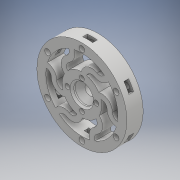
# Autodesk Inventor part: sea_ninjaflex
Saved by Autodesk Inventor 2018 (Build 220112000, 112)
## iProperties
Created: 2019-05-27
Part Number: sea_ninjaflex
Material: Generic
Document SubType Name: Modeling
Designer: Jasper
Mass: 17.2372 g
Surface Area: 57.8706 cm^2
Volume: 17.2372 cm^3
Density: 1 g/cm^3
Appearance: Default
Author: Jasper
Autodesk Inventor part; units mm, degrees
ref_plane "YZ Plane" through (0, 0, 0) normal (1, 0, 0) x (0, 1, 0)
ref_plane "XZ Plane" through (0, 0, 0) normal (0, 1, 0) x (-1, 0, 0)
sketch "Sketch1" plane through (0, 0, 0) normal (0, 1, 0) x (-1, 0, 0)
  circle A0 centre (0, 0) radius 25
  dimension "d0" = 50
  constraints: 1 centre point, 1 coincident
  measures "d0" diameter of A0
extrude "Extrusion1" add sketch "Sketch1" along normal blind 9
sketch "Sketch2" plane through (0, 9, 0) normal (0, 1, 0) x (1, 0, 0)
  line L0 (0, 0) -> (0, -22) construction
  line L1 (0, 0) -> (22, 0) construction
  circle A0 centre (0, -22) radius 1.6
  circle A1 centre (19.0526, -11) radius 1.6
  circle A2 centre (19.0526, 11) radius 1.6
  circle A3 centre (0, 22) radius 1.6
  circle A4 centre (-19.0526, 11) radius 1.6
  circle A5 centre (-19.0526, -11) radius 1.6
  dimension "d3" = 22
  dimension "d4" = 90
  dimension "d5" = 3.2
  dimension "d8" = 360
  constraints: 6 centre point, 4 end point, 1 coincident, 1 horizontal, 1 perpendicular, 1 vertical, 13 other
  measures "d3" distance of L0.start L0.end
  measures "d4" angle of L0 L1
  measures "d5" diameter of A0
extrude "Extrusion2" cut sketch "Sketch2" against normal up to surface (9 mm away)
ref_plane "Work Plane1" through (0, 3.2, 0) normal (0, 1, 0) x (1, 0, 0)
sketch "Sketch3" plane through (0, 3.2, 0) normal (0, 1, 0) x (1, 0, 0)
  circle A0 centre (-19.0526, 11) radius 1.6 construction
  circle A1 centre (-19.0526, -11) radius 1.6 construction
  circle A2 centre (0, 22) radius 1.6 construction
  circle A3 centre (19.0526, -11) radius 1.6 construction
  circle A4 centre (0, -22) radius 1.6 construction
  circle A5 centre (19.0526, 11) radius 1.6 construction
  circle A6 centre (0, 0) radius 25 construction
  line L0 (0, -25.2332) -> (-2.8, -23.6166)
  line L1 (-2.8, -23.6166) -> (-2.8, -20.3834)
  line L2 (-2.8, -20.3834) -> (0, -18.7668)
  line L3 (0, -18.7668) -> (2.8, -20.3834)
  line L4 (2.8, -20.3834) -> (2.8, -23.6166)
  line L5 (2.8, -23.6166) -> (0, -25.2332)
  line L6 (0, 0) -> (0, -18.7668)
  line L7 (0, 0) -> (18.7668, 0) construction
  line L8 (-2.8, -23.6166) -> (2.8, -23.6166)
  line L9 (2.8, -23.6166) -> (2.8, -26)
  line L10 (2.8, -26) -> (-2.8, -26)
  line L11 (-2.8, -26) -> (-2.8, -23.6166)
  line L12 (19.0526, -7.7668) -> (21.8526, -9.3834)
  line L13 (16.2526, -9.3834) -> (19.0526, -7.7668)
  line L14 (21.8526, -9.3834) -> (23.9167, -10.5751)
  line L15 (16.2526, -12.6166) -> (16.2526, -9.3834)
  line L16 (19.0526, -14.2332) -> (21.8526, -9.3834)
  line L17 (21.8526, -12.6166) -> (19.0526, -14.2332)
  line L18 (21.1167, -15.4249) -> (19.0526, -14.2332)
  line L19 (23.9167, -10.5751) -> (21.1167, -15.4249)
  line L20 (21.8526, -9.3834) -> (21.8526, -12.6166)
  line L21 (19.0526, -14.2332) -> (16.2526, -12.6166)
  line L22 (16.2526, 12.6166) -> (19.0526, 14.2332)
  line L23 (16.2526, 9.3834) -> (16.2526, 12.6166)
  line L24 (19.0526, 14.2332) -> (21.1167, 15.4249)
  line L25 (19.0526, 7.7668) -> (16.2526, 9.3834)
  line L26 (21.8526, 9.3834) -> (19.0526, 14.2332)
  line L27 (21.8526, 12.6166) -> (21.8526, 9.3834)
  line L28 (23.9167, 10.5751) -> (21.8526, 9.3834)
  line L29 (21.1167, 15.4249) -> (23.9167, 10.5751)
  line L30 (19.0526, 14.2332) -> (21.8526, 12.6166)
  line L31 (21.8526, 9.3834) -> (19.0526, 7.7668)
  line L32 (-2.8, 20.3834) -> (-2.8, 23.6166)
  line L33 (0, 18.7668) -> (-2.8, 20.3834)
  line L34 (-2.8, 23.6166) -> (-2.8, 26)
  line L35 (2.8, 20.3834) -> (0, 18.7668)
  line L36 (2.8, 23.6166) -> (-2.8, 23.6166)
  line L37 (0, 25.2332) -> (2.8, 23.6166)
  line L38 (2.8, 26) -> (2.8, 23.6166)
  line L39 (-2.8, 26) -> (2.8, 26)
  line L40 (-2.8, 23.6166) -> (0, 25.2332)
  line L41 (2.8, 23.6166) -> (2.8, 20.3834)
  line L42 (-19.0526, 7.7668) -> (-21.8526, 9.3834)
  line L43 (-16.2526, 9.3834) -> (-19.0526, 7.7668)
  line L44 (-21.8526, 9.3834) -> (-23.9167, 10.5751)
  line L45 (-16.2526, 12.6166) -> (-16.2526, 9.3834)
  line L46 (-19.0526, 14.2332) -> (-21.8526, 9.3834)
  line L47 (-21.8526, 12.6166) -> (-19.0526, 14.2332)
  line L48 (-21.1167, 15.4249) -> (-19.0526, 14.2332)
  line L49 (-23.9167, 10.5751) -> (-21.1167, 15.4249)
  line L50 (-21.8526, 9.3834) -> (-21.8526, 12.6166)
  line L51 (-19.0526, 14.2332) -> (-16.2526, 12.6166)
  line L52 (-16.2526, -12.6166) -> (-19.0526, -14.2332)
  line L53 (-16.2526, -9.3834) -> (-16.2526, -12.6166)
  line L54 (-19.0526, -14.2332) -> (-21.1167, -15.4249)
  line L55 (-19.0526, -7.7668) -> (-16.2526, -9.3834)
  line L56 (-21.8526, -9.3834) -> (-19.0526, -14.2332)
  line L57 (-21.8526, -12.6166) -> (-21.8526, -9.3834)
  line L58 (-23.9167, -10.5751) -> (-21.8526, -9.3834)
  line L59 (-21.1167, -15.4249) -> (-23.9167, -10.5751)
  line L60 (-19.0526, -14.2332) -> (-21.8526, -12.6166)
  line L61 (-21.8526, -9.3834) -> (-19.0526, -7.7668)
  point P0 (19.0526, 11)
  point P1 (0, 22)
  point P2 (-19.0526, 11)
  dimension "d13" = 5.6
  dimension "d14" = 90
  dimension "d15" = 5.6
  dimension "d16" = 2.3834
  dimension "d19" = 360
  constraints: 124 end point, 2 horizontal, 2 parallel, 2 perpendicular, 1 coincident, 134 other
  measures "d13" distance between parallel lines of L3 L0
  measures "d14" angle of L6 L7
  measures "d15" distance of L9.end L10.end
  measures "d16" distance between parallel lines of L10 L8
extrude "Extrusion3" cut sketch "Sketch3" along normal blind 2.6
sketch "Sketch4" plane through (0, 9, 0) normal (0, 1, 0) x (1, 0, 0)
  line L0 (0, 0) -> (8, 0) construction
  line L1 (0, 0) -> (8, 0) construction
  circle A0 centre (8, 0) radius 1.35
  circle A1 centre (0, 8) radius 1.35
  circle A2 centre (-8, 0) radius 1.35
  circle A3 centre (0, -8) radius 1.35
  dimension "d23" = 8
  dimension "d24" = 0
  dimension "d25" = 2.7
  dimension "d28" = 360
  constraints: 4 centre point, 4 end point, 2 horizontal, 1 coincident, 1 collinear, 9 other
  measures "d23" distance of L0.start L0.end
  measures "d24" distance between parallel lines of L0 L1
  measures "d25" diameter of A0
extrude "Extrusion4" cut sketch "Sketch4" against normal up to surface (9 mm away)
sketch "Sketch5" plane through (0, 9, 0) normal (0, 1, 0) x (1, 0, 0)
  circle A0 centre (-8, 0) radius 1.35 construction
  circle A1 centre (0, -8) radius 1.35 construction
  circle A2 centre (0, 8) radius 1.35 construction
  circle A3 centre (8, 0) radius 1.35 construction
  circle A4 centre (-19.0526, 11) radius 1.6 construction
  circle A5 centre (-19.0526, -11) radius 1.6 construction
  circle A6 centre (0, 22) radius 1.6 construction
  circle A7 centre (19.0526, -11) radius 1.6 construction
  circle A8 centre (0, -22) radius 1.6 construction
  circle A9 centre (19.0526, 11) radius 1.6 construction
  circle A10 centre (0, 0) radius 25 construction
  circle A11 centre (0, 8) radius 2.25
  circle A12 centre (-8, 0) radius 2.25
  circle A13 centre (0, -8) radius 2.25
  circle A14 centre (8, 0) radius 2.25
  dimension "d32" = 4.5
  dimension "d35" = 360
  constraints: 4 centre point, 1 coincident, 9 other
  measures "d32" diameter of A11
extrude "Extrusion5" cut sketch "Sketch5" against normal blind 5.5
sketch "Sketch6" plane through (0, 9, 0) normal (0, 1, 0) x (1, 0, 0)
  circle A0 centre (0, 0) radius 11
  dimension "d39" = 22
  constraints: 1 centre point, 1 coincident
  measures "d39" diameter of A0
extrude "Extrusion6" [suppressed]
sketch "Sketch7" plane through (0, 9, 0) normal (0, 1, 0) x (1, 0, 0)
  circle A0 centre (0, 0) radius 17.5 construction
  circle A1 centre (0, 0) radius 12.5 construction
  circle A2 centre (0, -8) radius 2.25 construction
  circle A3 centre (0, 8) radius 2.25 construction
  circle A4 centre (-8, 0) radius 2.25 construction
  circle A5 centre (8, 0) radius 2.25 construction
  circle A6 centre (-19.0526, 11) radius 1.6 construction
  circle A7 centre (-19.0526, -11) radius 1.6 construction
  circle A8 centre (0, 22) radius 1.6 construction
  circle A9 centre (19.0526, -11) radius 1.6 construction
  circle A10 centre (0, -22) radius 1.6 construction
  circle A11 centre (19.0526, 11) radius 1.6 construction
  circle A12 centre (0, 0) radius 25 construction
  line L0 (0.0443, -12.4999) -> (-1.2042, -12.4373)
  line L1 (0.0443, -12.4999) -> (1.2943, -12.4999) construction
  line L2 (0.0443, -12.4999) -> (1.2927, -12.4373)
  line L3 (0.0443, -12.4999) -> (1.2943, -12.4999) construction
  line L4 (-1.2042, -12.4373) -> (3.5115, -17.153)
  line L5 (-1.2042, -12.4373) -> (5.4648, -12.4373) construction
  line L6 (1.2796, -12.4428) -> (5.4791, -16.6424)
  line L7 (1.2796, -12.4428) -> (7.2186, -12.4428) construction
  arc A13 (-1.1991, -12.4423) -> (1.2796, -12.4428) centre (0.0427, -0.0042) ccw
  arc A14 (3.5115, -17.153) -> (5.4791, -16.6424) centre (0.1064, 0.0125) ccw
  line L8 (3.6487, -11.9681) -> (9.8101, -14.5202)
  arc A15 (3.6553, -11.9708) -> (5.9455, -11.0227) centre (0.0427, -0.0042) ccw
  line L9 (5.9455, -11.0227) -> (11.4325, -13.2954)
  arc A16 (9.8101, -14.5202) -> (11.4325, -13.2954) centre (0.0952, 0.0356) ccw
  line L10 (7.9526, -9.6774) -> (14.6216, -9.6774)
  arc A17 (7.9597, -9.6774) -> (9.7128, -7.925) centre (0.0427, -0.0042) ccw
  line L11 (9.7128, -7.925) -> (15.6518, -7.925)
  arc A18 (14.6216, -9.6774) -> (15.6518, -7.925) centre (0.076, 0.0526) ccw
  line L12 (11.0523, -5.9141) -> (17.2136, -3.362)
  arc A19 (11.0588, -5.9114) -> (12.0079, -3.6215) centre (0.0427, -0.0042) ccw
  line L13 (12.0079, -3.6215) -> (17.4948, -1.3488)
  arc A20 (17.2136, -3.362) -> (17.4948, -1.3488) centre (0.0517, 0.061) ccw
  line L14 (12.4759, -1.2511) -> (17.1916, 3.4646)
  arc A21 (12.4809, -1.2461) -> (12.4814, 1.2327) centre (0.0427, -0.0042) ccw
  line L15 (12.4814, 1.2327) -> (16.6809, 5.4322)
  arc A22 (17.1916, 3.4646) -> (16.6809, 5.4322) centre (0.026, 0.0595) ccw
  line L16 (12.0066, 3.6018) -> (14.5587, 9.7631)
  arc A23 (12.0093, 3.6083) -> (11.0612, 5.8986) centre (0.0427, -0.0042) ccw
  line L17 (11.0612, 5.8986) -> (13.334, 11.3855)
  arc A24 (14.5587, 9.7631) -> (13.334, 11.3855) centre (0.0029, 0.0483) ccw
  line L18 (9.716, 7.9057) -> (9.716, 14.5747)
  arc A25 (9.716, 7.9128) -> (7.9636, 9.6659) centre (0.0427, -0.0042) ccw
  line L19 (7.9636, 9.6659) -> (7.9636, 15.6049)
  arc A26 (9.716, 14.5747) -> (7.9636, 15.6049) centre (-0.0141, 0.029) ccw
  line L20 (5.9527, 11.0054) -> (3.4005, 17.1667)
  arc A27 (5.9499, 11.0119) -> (3.6601, 11.961) centre (0.0427, -0.0042) ccw
  line L21 (3.6601, 11.961) -> (1.3873, 17.4479)
  arc A28 (3.4005, 17.1667) -> (1.3873, 17.4479) centre (-0.0225, 0.0048) ccw
  line L22 (1.2896, 12.4289) -> (-3.4261, 17.1446)
  arc A29 (1.2846, 12.434) -> (-1.1942, 12.4345) centre (0.0427, -0.0042) ccw
  line L23 (-1.1942, 12.4345) -> (-5.3937, 16.634)
  arc A30 (-3.4261, 17.1446) -> (-5.3937, 16.634) centre (-0.0209, -0.0209) ccw
  line L24 (-3.5633, 11.9597) -> (-9.7246, 14.5118)
  arc A31 (-3.5698, 11.9624) -> (-5.8601, 11.0143) centre (0.0427, -0.0042) ccw
  line L25 (-5.8601, 11.0143) -> (-11.347, 13.287)
  arc A32 (-9.7246, 14.5118) -> (-11.347, 13.287) centre (-0.0097, -0.044) ccw
  line L26 (-7.8671, 9.669) -> (-14.5361, 9.669)
  arc A33 (-7.8742, 9.669) -> (-9.6273, 7.9166) centre (0.0427, -0.0042) ccw
  line L27 (-9.6273, 7.9166) -> (-15.5663, 7.9166)
  arc A34 (-14.5361, 9.669) -> (-15.5663, 7.9166) centre (0.0095, -0.061) ccw
  line L28 (-10.9668, 5.9057) -> (-17.1282, 3.3536)
  arc A35 (-10.9734, 5.903) -> (-11.9224, 3.6131) centre (0.0427, -0.0042) ccw
  line L29 (-11.9224, 3.6131) -> (-17.4093, 1.3404)
  arc A36 (-17.1282, 3.3536) -> (-17.4093, 1.3404) centre (0.0338, -0.0694) ccw
  line L30 (-12.3904, 1.2427) -> (-17.1061, -3.473)
  arc A37 (-12.3954, 1.2377) -> (-12.3959, -1.2411) centre (0.0427, -0.0042) ccw
  line L31 (-12.3959, -1.2411) -> (-16.5954, -5.4406)
  arc A38 (-17.1061, -3.473) -> (-16.5954, -5.4406) centre (0.0594, -0.0679) ccw
  line L32 (-11.9212, -3.6102) -> (-14.4733, -9.7715)
  arc A39 (-11.9239, -3.6167) -> (-10.9757, -5.907) centre (0.0427, -0.0042) ccw
  line L33 (-10.9757, -5.907) -> (-13.2485, -11.3939)
  arc A40 (-14.4733, -9.7715) -> (-13.2485, -11.3939) centre (0.0825, -0.0566) ccw
  line L34 (-9.6305, -7.9141) -> (-9.6305, -14.5831)
  arc A41 (-9.6305, -7.9212) -> (-7.8781, -9.6743) centre (0.0427, -0.0042) ccw
  line L35 (-7.8781, -9.6743) -> (-7.8781, -15.6133)
  arc A42 (-9.6305, -14.5831) -> (-7.8781, -15.6133) centre (0.0996, -0.0374) ccw
  line L36 (-5.8672, -11.0138) -> (-3.3151, -17.1751)
  arc A43 (-5.8645, -11.0203) -> (-3.5746, -11.9694) centre (0.0427, -0.0042) ccw
  line L37 (-3.5746, -11.9694) -> (-1.3018, -17.4563)
  arc A44 (-3.3151, -17.1751) -> (-1.3018, -17.4563) centre (0.1079, -0.0131) ccw
  dimension "d42" = 35
  dimension "d43" = 25
  dimension "d46" = 1.25
  dimension "d47" = 177.13
  dimension "d48" = 1.25
  dimension "d49" = 2.87
  dimension "d50" = 6.669
  dimension "d51" = 45
  dimension "d52" = 5.939
  dimension "d53" = 45
  dimension "d54" = 12.5
  dimension "d55" = 17.5
  dimension "d58" = 360
  constraints: 76 end point, 66 point on circle, 34 centre point, 16 point on line, 4 coincident, 4 equal length, 4 horizontal, 175 other
  measures "d42" diameter of A0
  measures "d43" diameter of A1
  measures "d46" distance of L0.start L0.end
  measures "d47" angle of L1 L0
  measures "d48" distance of L0.start L2.end
  measures "d49" angle of L3 L2
  measures "d50" distance of L0.end L4.end
  measures "d51" angle of L4 L5
  measures "d52" distance of L6.start L6.end
  measures "d53" angle of L6 L7
  measures "d54" radius of A13
  measures "d55" radius of A14
extrude "Extrusion7" [suppressed]
sketch "Sketch9" plane through (0, 0, 0) normal (0, -1, 0) x (1, 0, 0)
  circle A0 centre (0, 0) radius 5.5
  dimension "d63" = 11
  constraints: 1 centre point, 1 coincident
  measures "d63" diameter of A0
extrude "Extrusion8" cut sketch "Sketch9" against normal blind 1.8
sketch "Sketch10" plane through (0, 1.8, 0) normal (0, -1, 0) x (1, 0, 0)
  circle A0 centre (0, 0) radius 2.8
  dimension "d66" = 5.6
  constraints: 1 centre point, 1 coincident
  measures "d66" diameter of A0
extrude "Extrusion9" cut sketch "Sketch10" against normal up to surface (7.2 mm away)
chamfer "Chamfer1" distance 1 angle 45 1 edges at (-5.5, 0, 0)
chamfer "Chamfer2" distance 2.7 angle 45 1 edges at (-2.8, 1.8, 0)
sketch "Sketch11" plane through (0, 9, 0) normal (0, 1, 0) x (1, 0, 0)
  circle A0 centre (0, 0) radius 20 construction
  circle A1 centre (0, 0) radius 11
  circle A2 centre (0, -8) radius 2.25 construction
  circle A3 centre (0, 8) radius 2.25 construction
  circle A4 centre (-8, 0) radius 2.25 construction
  circle A5 centre (8, 0) radius 2.25 construction
  circle A6 centre (-19.0526, 11) radius 1.6 construction
  circle A7 centre (-19.0526, -11) radius 1.6 construction
  circle A8 centre (0, 22) radius 1.6 construction
  circle A9 centre (19.0526, -11) radius 1.6 construction
  circle A10 centre (0, -22) radius 1.6 construction
  circle A11 centre (19.0526, 11) radius 1.6 construction
  circle A12 centre (0, 0) radius 25 construction
  line L0 (20, 0) -> (8, 0) construction
  arc A13 (19.775, 2.9916) -> (17, 0) centre (20, 0) ccw
  arc A14 (19.1, 5.9321) -> (14, 0) centre (20, 0) ccw
  arc A15 (9.3636, -5.7725) -> (17, 0) centre (11, 0) ccw
  arc A16 (10.5909, -2.972) -> (14, 0) centre (11, 0) ccw
  arc A17 (19.775, 2.9916) -> (19.1, 5.9321) centre (0, 0) ccw
  line L1 (0, 0) -> (11, 0) construction
  line L2 (0, 0) -> (11, 0) construction
  arc A18 (10.5909, -2.972) -> (11, 0) centre (0, 0) ccw construction
  line L3 (0, 0) -> (11, 0) construction
  line L4 (0, 0) -> (11, 0) construction
  arc A19 (9.3636, -5.7725) -> (10.5909, -2.972) centre (0, 0) ccw
  line L5 (0, 0) -> (20, 0) construction
  arc A20 (4.4126, 19.5071) -> (7, 12.1244) centre (10, 17.3205) ccw
  arc A21 (7.8693, 7.686) -> (7, 12.1244) centre (5.5, 9.5263) ccw
  arc A22 (9.681, 5.2229) -> (7.8693, 7.686) centre (0, 0) ccw
  arc A23 (9.681, 5.2229) -> (8.5, 14.7224) centre (5.5, 9.5263) ccw
  arc A24 (7.2967, 18.6214) -> (8.5, 14.7224) centre (10, 17.3205) ccw
  arc A25 (7.2967, 18.6214) -> (4.4126, 19.5071) centre (0, 0) ccw
  arc A26 (-14.6874, 13.575) -> (-7, 12.1244) centre (-10, 17.3205) ccw
  arc A27 (-2.7216, 10.658) -> (-7, 12.1244) centre (-5.5, 9.5263) ccw
  arc A28 (0.3174, 10.9954) -> (-2.7216, 10.658) centre (0, 0) ccw
  arc A29 (0.3174, 10.9954) -> (-8.5, 14.7224) centre (-5.5, 9.5263) ccw
  arc A30 (-12.4783, 15.6299) -> (-8.5, 14.7224) centre (-10, 17.3205) ccw
  arc A31 (-12.4783, 15.6299) -> (-14.6874, 13.575) centre (0, 0) ccw
  arc A32 (-19.1, -5.9321) -> (-14, 0) centre (-20, 0) ccw
  arc A33 (-10.5909, 2.972) -> (-14, 0) centre (-11, 0) ccw
  arc A34 (-9.3636, 5.7725) -> (-10.5909, 2.972) centre (0, 0) ccw
  arc A35 (-9.3636, 5.7725) -> (-17, 0) centre (-11, 0) ccw
  arc A36 (-19.775, -2.9916) -> (-17, 0) centre (-20, 0) ccw
  arc A37 (-19.775, -2.9916) -> (-19.1, -5.9321) centre (0, 0) ccw
  arc A38 (-4.4126, -19.5071) -> (-7, -12.1244) centre (-10, -17.3205) ccw
  arc A39 (-7.8693, -7.686) -> (-7, -12.1244) centre (-5.5, -9.5263) ccw
  arc A40 (-9.681, -5.2229) -> (-7.8693, -7.686) centre (0, 0) ccw
  arc A41 (-9.681, -5.2229) -> (-8.5, -14.7224) centre (-5.5, -9.5263) ccw
  arc A42 (-7.2967, -18.6214) -> (-8.5, -14.7224) centre (-10, -17.3205) ccw
  arc A43 (-7.2967, -18.6214) -> (-4.4126, -19.5071) centre (0, 0) ccw
  arc A44 (14.6874, -13.575) -> (7, -12.1244) centre (10, -17.3205) ccw
  arc A45 (2.7216, -10.658) -> (7, -12.1244) centre (5.5, -9.5263) ccw
  arc A46 (-0.3174, -10.9954) -> (2.7216, -10.658) centre (0, 0) ccw
  arc A47 (-0.3174, -10.9954) -> (8.5, -14.7224) centre (5.5, -9.5263) ccw
  arc A48 (12.4783, -15.6299) -> (8.5, -14.7224) centre (10, -17.3205) ccw
  arc A49 (12.4783, -15.6299) -> (14.6874, -13.575) centre (0, 0) ccw
  arc A50 (10.5909, -2.972) -> (9.681, 5.2229) centre (0, 0) ccw construction
  arc A51 (19.1877, 5.1593) -> (19.1, 5.475) centre (0, 0) ccw construction
  arc A52 (19.1, 5.9321) -> (7.2967, 18.6214) centre (0, 0) ccw construction
  arc A53 (10.5909, -2.972) -> (9.681, 5.2229) centre (0, 0) ccw
  arc A54 (19.1, 5.9321) -> (7.2967, 18.6214) centre (0, 0) ccw
  dimension "d19" = 360
  dimension "d76" = 22
  dimension "d75" = 40
  dimension "d79" = 12
  dimension "d83" = 3
  dimension "d84" = 6
  dimension "d85" = 11
  dimension "d86" = 360
  dimension "d87" = 11
  dimension "d88" = 0
  dimension "d91" = 360
  constraints: 87 point on circle, 43 centre point, 25 coincident, 12 end point, 3 collinear, 2 horizontal, 2 point on line, 1 horizontal alignment, 1 midpoint, 109 other
  measures "d75" diameter of A0
  measures "d79" distance of L0.start L0.end
  measures "d83" radius of A13
  measures "d84" radius of A14
  measures "d85" distance of L1.start L1.end
  measures "d87" radius of A18
  measures "d88" distance between parallel lines of L3 L4
extrude "Extrusion10" cut sketch "Sketch11" against normal through all contours A1 A23 A24 A54 A14 A16
pattern_circular "Circular Pattern1" count 6 over 360 about axis through (0, -10, 0) along (0, 1, 0) of "Extrusion10"
equation "\"alpha\" = 45deg"
body "Solid1"
